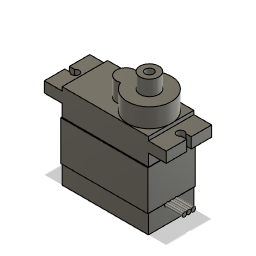
CAM v42 (Autodesk Fusion 360 archive; units mm, degrees)
design "MG90_Rebuild"
Autodesk Fusion 360 part; units mm, degrees
note: some values were not read from the file. Chosen so that the rebuilt part matches the saved one: which face or edge a step refers to. Set by a fixed rule: which sketch regions a step uses.
sketch "ServoRotatingPlate" plane through (0, 0, 0) normal (0, 1, 0) x (1, 0, 0)
  circle A0 centre (0, 0) radius 5.8
  line L0 (5.75, 6) -> (-17.05, 6)
  line L1 (-17.05, 6) -> (-17.05, -6)
  line L2 (-17.05, -6) -> (5.75, -6)
  line L3 (5.75, -6) -> (5.75, 6)
  line L4 (-8.7, 0) -> (5.75, 0) construction
  circle A1 centre (-6.2, 0) radius 2.5
  circle A2 centre (0, 0) radius 2.5
  circle A3 centre (0, 0) radius 1.1
  point P0 (5.8, 0)
  dimension "d4" = 11.6
  dimension "d6" = 12
  dimension "d7" = 22.8
  dimension "d10" = 5
  dimension "d12" = 14.5
  dimension "d13" = 5.75
  dimension "d14" = 8.35
  dimension "d48" = 5
  dimension "d49" = 1.4
  constraint coincident A0.centre A2.centre
  constraint horizontal L0
  constraint vertical L1
  constraint horizontal L2
  constraint vertical L3
  constraint horizontal L4
  constraint midpoint L3 L4.end
  constraint coincident L4 A1.centre
  constraint coincident L4.start A1
  constraint coincident A0.centre L4
  constraint coincident L4 P0
  constraint coincident A0 P0
  constraint concentric A0 A2
  constraint concentric A2 A3
  measures "d4" diameter of A0
  measures "d6" distance of L0.start L2.end
  measures "d7" distance of L0.start L0.end
  measures "d10" diameter of A1
  measures "d12" distance of L4.start P0
  measures "d13" distance of A0.centre L3
  measures "d14" distance of L1 L4.start
  measures "d48" diameter of A2
  measures "d49" distance of A2 A3
extrude "Extrude1" add sketch "ServoRotatingPlate" against normal blind 5 contours A0 L3 | A0 L3 A1 | A0 A1 | A0 A1 | A2 | A3
extrude "Extrude2" add sketch "ServoRotatingPlate" against normal blind 22.5 from surface at -5 contours A0 L3 A1 | A0 L0 L1 L2 L3 A1 | A0 A1 | A0 A1 | A2 | A3
ref_plane "WorkPlane1" through (-5.65, -6, 0) normal (0, 1, 0) x (0, 0, 1)
sketch "EarBase" plane through (-5.65, -6, 0) normal (0, 1, 0) x (1, 0, 0)
  line L0 (16.1, 6) -> (-16.1, 6)
  line L1 (-16.1, 6) -> (-16.1, -6)
  line L2 (-16.1, -6) -> (16.1, -6)
  line L3 (16.1, -6) -> (16.1, 6)
  line L4 (16.1, 6) -> (-16.1, -6) construction
  line L5 (-16.1, 6) -> (16.1, -6) construction
  line L6 (-16.1, 0) -> (16.1, 0) construction
  circle A0 centre (-13.9, 0) radius 1
  line L7 (-14.7, 0.6) -> (-16.1, 0.6)
  line L8 (-14.7, -0.6) -> (-16.1, -0.6)
  line L9 (-11.4, 6) -> (-11.4, -6)
  line L10 (0, 0) -> (0, 6) construction
  line L11 (14.7, 0.6) -> (16.1, 0.6)
  circle A1 centre (13.9, 0) radius 1
  line L12 (14.7, -0.6) -> (16.1, -0.6)
  point P0 (11.4, 6)
  dimension "d26" = 32.2
  dimension "d31" = 2
  dimension "d33" = 1.2
  dimension "d34" = 2.5
  dimension "d35" = 4.7
  constraint perpendicular L0 L1
  constraint parallel L0 L2
  constraint parallel L1 L3
  constraint horizontal L0
  constraint coincident L4 L10.start
  constraint coincident L5 L10.start
  constraint coincident L10.start origin
  constraint coincident L0 P0
  constraint midpoint L1 L6.start
  constraint midpoint L3 L6.end
  constraint coincident L6 A0.centre
  constraint coincident A0 L7.start
  constraint coincident L1 L7.end
  constraint perpendicular L1 L7
  constraint symmetric L6 L7.start L8.start
  constraint symmetric L6 L7.end L8.end
  constraint midpoint L0 L10.end
  constraint symmetric A0 L10 A1
  constraint symmetric L7.start L10 L11.start
  constraint symmetric L7.end L10 L11.end
  constraint symmetric L8.start L10 L12.start
  constraint symmetric L8.end L10 L12.end
  measures "d26" distance of L0.start L0.end
  measures "d31" diameter of A0
  measures "d33" distance of L7.end L8.end
  measures "d34" distance of A0.centre L9
  measures "d35" distance of L0.end L9.start
extrude "Extrude3" add sketch "EarBase" against normal blind 2.8 contours L0 L2 L3 L9 L11 A1 L12 | L0 L1 L2 A0 L7 L8 L9
ref_plane "WorkPlane2" through (-5.65, -22.5, 0) normal (0, -1, 0) x (0, 0, -1)
sketch "StickerBase" plane through (-5.65, -22.5, 0) normal (0, -1, 0) x (1, 0, 0)
  line L0 (11.5, -6.25) -> (-11.5, -6.25)
  line L1 (-11.5, -6.25) -> (-11.5, 6.25)
  line L2 (-11.5, 6.25) -> (11.5, 6.25)
  line L3 (11.5, 6.25) -> (11.5, -6.25)
  line L4 (11.5, -6.25) -> (-11.5, 6.25) construction
  line L5 (-11.5, -6.25) -> (11.5, 6.25) construction
  dimension "d42" = 23
  dimension "d43" = 12.5
  constraint perpendicular L0 L1
  constraint parallel L0 L2
  constraint parallel L1 L3
  constraint horizontal L0
  constraint coincident L4 origin
  constraint coincident L5 origin
  measures "d42" distance of L0.start L0.end
  measures "d43" distance of L0.start L2.end
extrude "Extrude4" add sketch "StickerBase" against normal blind 10.5
extrude "Extrude5" add sketch "ServoRotatingPlate" along normal blind 4 contours A2
sketch "WireHardCoded" plane through (5.75, 0, 0) normal (1, 0, 0) x (0, 0, -1)
  line L0 (6, -22.5) -> (-6, -22.5)
  line L1 (-6, -22.5) -> (-6, -27.5)
  line L2 (-6, -27.5) -> (6, -27.5)
  line L3 (6, -27.5) -> (6, -22.5)
  line L4 (-1.75, -23.5) -> (1.75, -23.5) construction
  line L5 (1.75, -23.5) -> (1.75, -22.3333) construction
  line L6 (1.75, -22.3333) -> (-1.75, -22.3333) construction
  line L7 (-1.75, -22.3333) -> (-1.75, -23.5) construction
  line L8 (0, -27.5) -> (0, -23.5) construction
  line L9 (-1.75, -22.9167) -> (1.75, -22.9167) construction
  circle A0 centre (0, -22.9167) radius 0.5833
  circle A1 centre (-1.17, -22.9167) radius 0.5833
  circle A2 centre (1.17, -22.9167) radius 0.5833
  dimension "d52" = 1.1667
  dimension "d53" = 3.5
  dimension "d54" = 4
  dimension "d57" = 1.17
  dimension "d58" = 0
  constraint horizontal L4
  constraint vertical L5
  constraint horizontal L6
  constraint vertical L7
  constraint midpoint L2 L8.start
  constraint midpoint L4 L8.end
  constraint vertical L8
  constraint midpoint L7 L9.start
  constraint midpoint L5 L9.end
  constraint midpoint L9 A0.centre
  constraint tangent L6 A0
  measures "d52" distance of L4.end L5.end
  measures "d53" distance of L4.start L4.end
  measures "d54" distance of L8.start L8.end
extrude "Extrude6" add sketch "WireHardCoded" along normal up to surface (4.7 mm away) contours L0 A2 | L0 A2 | L0 A0 | L0 A0 | L0 A1 | L0 A1
equation "Note0 = 0" comment "The [0,0,0] is placed at the servo shaft base plane, for better alignment"
equation "Note1 = 1" comment "Improvement for https://www.thingiverse.com/thing:2641076"
equation "BaseCircleD = 11.6 mm"
equation "d4 = BaseCircleD"
equation "BaseRectW = 12 mm"
equation "d6 = BaseRectW"
equation "d7 = BaseRectH"
equation "BaseRectH = 22.8 mm"
equation "BaseCircle2D = 5 mm"
equation "d10 = BaseCircle2D"
equation "E2EDist = 14.5 mm"
equation "d12 = E2EDist"
equation "d13 = CenterMeasureL"
equation "CenterMeasureL = 5.75 mm"
equation "GearIsleHeight = 5 mm"
equation "d17 = -GearIsleHeight"
equation "BoxHeight = 22.5 mm"
equation "d21 = -BoxHeight"
equation "Ear_Down = 1 mm"
equation "d24 = -Ear_Down"
equation "Ear_L = 32.2 mm"
equation "d26 = Ear_L"
equation "Ear_Thick = 2.8 mm"
equation "d28 = -Ear_Thick"
equation "EarScrew_D = 2 mm"
equation "d31 = EarScrew_D"
equation "Ear_Slit = 1.2 mm"
equation "d33 = Ear_Slit"
equation "d34 = HolePos"
equation "HolePos = 2.5 mm"
equation "sticker_height = 10.5 mm"
equation "stick_pos = 5 mm"
equation "d39 = -stick_pos"
equation "Sticker_Profile_L = 23 mm"
equation "Sticker_Profile_W = 12.5 mm"
equation "d42 = Sticker_Profile_L"
equation "d43 = Sticker_Profile_W"
equation "d44 = -sticker_height"
equation "ServoShaftProf = 5 mm"
equation "ServoProfHeight = 4 mm"
equation "d48 = ServoShaftProf"
equation "d50 = ServoProfHeight"
equation "d52 = ( 3.5 / 3 ) * 1 mm"
named bodies: "WireHardCoded"

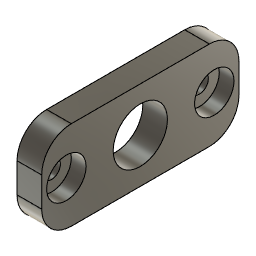
design "mil_tutucu"
Autodesk Fusion 360 part; units mm, degrees
sketch "Sketch1" plane through (0, 0, 0) normal (1, 0, 0) x (0, 1, 0)
  line L0 (0, 0) -> (40, 0)
  line L1 (40, 0) -> (40, 18)
  line L2 (40, 18) -> (0, 18)
  line L3 (0, 18) -> (0, 0)
  circle A0 centre (20, 9) radius 5.5
  line L4 (0, 9) -> (40, 9) construction
  dimension "d1" = 18
  dimension "d2" = 40
  dimension "d3" = 11
  constraint horizontal L0
  constraint vertical L1
  constraint horizontal L2
  constraint vertical L3
  constraint coincident L0.start L3.end
  constraint midpoint L3 L4.start
  constraint midpoint L1 L4.end
  constraint midpoint A0.centre L4
  measures "d1" distance of L0.end L1.end
  measures "d2" distance of L1.end L2.end
  measures "d3" diameter of A0
extrude "Extrude1" add sketch "Sketch1" along normal blind 5
fillet "Fillet1" radius 6 4 edges at (2.5, 0, 18) (2.5, 0, 0) (2.5, 40, 0) (2.5, 40, 18)
sketch "Sketch2" plane through (5, 0, 0) normal (1, 0, 0) x (0, 1, 0)
  circle A0 centre (20, 9) radius 5.5
  arc A1 (40, 12) -> (34, 18) centre (34, 12) ccw
  line L0 (34, 18) -> (6, 18)
  arc A2 (6, 18) -> (0, 12) centre (6, 12) ccw
  line L1 (0, 12) -> (0, 6)
  arc A3 (0, 6) -> (6, 0) centre (6, 6) ccw
  line L2 (6, 0) -> (34, 0)
  arc A4 (34, 0) -> (40, 6) centre (34, 6) ccw
  line L3 (40, 6) -> (40, 12)
  line L4 (40, 9) -> (0, 9) construction
  point P0 (5, 9)
  point P1 (35, 9)
  dimension "d8" = 5
  dimension "d9" = 5
  constraint horizontal P0 P1
  constraint midpoint L3 L4.start
  constraint midpoint L1 L4.end
  constraint coincident P1 L4
  measures "d8" distance of P1 L4.start
  measures "d9" distance of P0 L4.end
hole "Hole1" at (5, 5, 9) at (5, 35, 9) direction (-1, 0, 0) diameter 3.6 depth 7 tip angle 118 counterbore diameter 8 counterbore depth 3

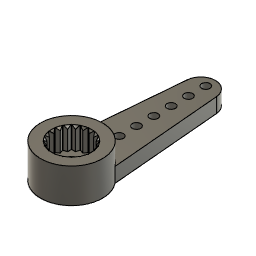
design "MG90_Arm"
Autodesk Fusion 360 part; units mm, degrees
sketch "Arm01Base" plane through (0, 0, 0) normal (0, 1, 0) x (1, 0, 0)
  circle A0 centre (0, 0) radius 3.7
  circle A1 centre (0, 0) radius 2.7
  line L0 (0, -3.7) -> (0, 17.2) construction
  circle A2 centre (0, 15.45) radius 1.75
  line L1 (-1.7434, 15.6016) -> (-2.9, 2.2978)
  line L2 (1.7434, 15.6016) -> (2.9, 2.2978)
  circle A3 centre (0, 0) radius 1.375
  circle A4 centre (0, 16.05) radius 0.5
  circle A5 centre (0, 13.98) radius 0.5
  circle A6 centre (0, 11.91) radius 0.5
  circle A7 centre (0, 9.84) radius 0.5
  circle A8 centre (0, 7.77) radius 0.5
  circle A9 centre (0, 5.7) radius 0.5
  point P0 (0, 16.55)
  dimension "d2" = 7.4
  dimension "d3" = 1
  dimension "d4" = 20.9
  dimension "d5" = 3.5
  dimension "d6" = 2.9
  dimension "d7" = 2.75
  dimension "d8" = 1
  dimension "d9" = 0.65
  dimension "d12" = 0
  dimension "d13" = -10.35
  constraint coincident A0.centre A1.centre
  constraint coincident A0 L0.start
  constraint vertical L0
  constraint coincident A0.centre L0
  constraint coincident L0 A2.centre
  constraint coincident L0.end A2
  constraint coincident A2 L1.start
  constraint coincident A0 L1.end
  constraint tangent A2 L1
  constraint symmetric L0 L1.start L2.start
  constraint symmetric L0 L1.end L2.end
  constraint concentric A1 A3
  constraint coincident L0 A4.centre
  constraint coincident A4 P0
  constraint coincident L0 P0
  measures "d2" diameter of A0
  measures "d3" distance of A0 A1
  measures "d4" distance of L0.start L0.end
  measures "d5" diameter of A2
  measures "d6" distance of L0 L1.end
  measures "d7" diameter of A3
  measures "d8" diameter of A4
  measures "d9" distance of L0.end P0
extrude "Extrude1" add sketch "Arm01Base" along normal blind 1.75 contours A0 | A0 A2 L1 L2 A5 | A2 A5 picked at (0.7406, 14.9094) makes body 1
extrude "Extrude2" add sketch "Arm01Base" along normal blind 4.1 contours A0 bodies 1
ref_plane "WorkPlane1" through (0, 1.5, 0) normal (0, 1, 0) x (0, 0, 1)
extrude "Extrude3" add sketch "Arm01Base" against normal blind 0.5 from surface at 1.5 contours A1 bodies 1
sketch "Teeth01" plane through (0, 1.5, 0) normal (0, 1, 0) x (1, 0, 0)
  circle A0 centre (0, 0) radius 2.1 construction
  circle A1 centre (0, 0) radius 2.4 construction
  line L0 (0, 0) -> (0, 2.4) construction
  line L1 (-0.35, 2.3743) -> (0, 2.1)
  line L2 (0.35, 2.3743) -> (0, 2.1)
  line L3 (-1.0666, 2.15) -> (-0.6489, 1.9972)
  line L4 (-0.4008, 2.3663) -> (-0.6489, 1.9972)
  line L5 (-1.6788, 1.7152) -> (-1.2343, 1.6989)
  line L6 (-1.1124, 2.1266) -> (-1.2343, 1.6989)
  line L7 (-2.1266, 1.1124) -> (-1.6989, 1.2343)
  line L8 (-1.7152, 1.6788) -> (-1.6989, 1.2343)
  line L9 (-2.3663, 0.4008) -> (-1.9972, 0.6489)
  line L10 (-2.15, 1.0666) -> (-1.9972, 0.6489)
  line L11 (-2.3743, -0.35) -> (-2.1, 0)
  line L12 (-2.3743, 0.35) -> (-2.1, 0)
  line L13 (-2.15, -1.0666) -> (-1.9972, -0.6489)
  line L14 (-2.3663, -0.4008) -> (-1.9972, -0.6489)
  line L15 (-1.7152, -1.6788) -> (-1.6989, -1.2343)
  line L16 (-2.1266, -1.1124) -> (-1.6989, -1.2343)
  line L17 (-1.1124, -2.1266) -> (-1.2343, -1.6989)
  line L18 (-1.6788, -1.7152) -> (-1.2343, -1.6989)
  line L19 (-0.4008, -2.3663) -> (-0.6489, -1.9972)
  line L20 (-1.0666, -2.15) -> (-0.6489, -1.9972)
  line L21 (0.35, -2.3743) -> (0, -2.1)
  line L22 (-0.35, -2.3743) -> (0, -2.1)
  line L23 (1.0666, -2.15) -> (0.6489, -1.9972)
  line L24 (0.4008, -2.3663) -> (0.6489, -1.9972)
  line L25 (1.6788, -1.7152) -> (1.2343, -1.6989)
  line L26 (1.1124, -2.1266) -> (1.2343, -1.6989)
  line L27 (2.1266, -1.1124) -> (1.6989, -1.2343)
  line L28 (1.7152, -1.6788) -> (1.6989, -1.2343)
  line L29 (2.3663, -0.4008) -> (1.9972, -0.6489)
  line L30 (2.15, -1.0666) -> (1.9972, -0.6489)
  line L31 (2.3743, 0.35) -> (2.1, 0)
  line L32 (2.3743, -0.35) -> (2.1, 0)
  line L33 (2.15, 1.0666) -> (1.9972, 0.6489)
  line L34 (2.3663, 0.4008) -> (1.9972, 0.6489)
  line L35 (1.7152, 1.6788) -> (1.6989, 1.2343)
  line L36 (2.1266, 1.1124) -> (1.6989, 1.2343)
  line L37 (1.1124, 2.1266) -> (1.2343, 1.6989)
  line L38 (1.6788, 1.7152) -> (1.2343, 1.6989)
  line L39 (0.4008, 2.3663) -> (0.6489, 1.9972)
  line L40 (1.0666, 2.15) -> (0.6489, 1.9972)
  circle A2 centre (0, 0) radius 2.7
  circle A3 centre (0, 0) radius 2.4
  dimension "d22" = 4.2
  dimension "d23" = 4.8
  dimension "d24" = 0.35
  dimension "d26" = 360
  constraint coincident A0.centre A1.centre
  constraint concentric A0 A1
  constraint coincident A1 L0.end
  constraint vertical L0
  constraint coincident A1 L1.start
  constraint coincident A0 L1.end
  constraint coincident L0 L1.end
  constraint coincident A1 L2.start
  constraint symmetric L0 L1.start L2.start
  constraint coincident L39.start A3
  measures "d22" diameter of A0
  measures "d23" diameter of A1
  measures "d24" horizontal distance of L0.end L2.start
extrude "Extrude4" add sketch "Teeth01" along normal up to surface (2.6 mm away) contours L1 L2 A3 | L3 L4 A3 | L39 L40 A3 | L5 L6 A3 | L37 L38 A3 | L7 L8 A3 | L35 L36 A3 | L9 L10 A3 | L33 L34 A3 | L11 L12 A3 | L31 L32 A3 | L13 L14 A3 | L29 L30 A3 | L15 L16 A3 | L27 L28 A3 | L17 L18 A3 | L25 L26 A3 | L19 L20 A3 | L23 L24 A3 | L21 L22 A3 | A2 bodies 1
sketch "TeethChamfer01" plane through (0, 0, 0) normal (1, 0, 0) x (0, 0, -1)
  line L0 (3.7, 4.1) -> (-3.7, 4.1) construction
  line L1 (0, 0) -> (0, 4.1) construction
  line L2 (2.3743, 4.1) -> (2.1, 3.8)
  line L3 (2.1, 3.8) -> (2.1, 4.1)
  line L4 (2.3743, 4.1) -> (2.1, 4.1)
  point P0 (2.3743, 4.1)
  point P1 (2.1, 4.1)
  dimension "d29" = 0.3
  constraint coincident L1.start origin
  constraint midpoint L0 L1.end
  constraint coincident P0 L2.start
  constraint coincident L0 P1
  constraint perpendicular L0 L3
  constraint coincident P1 L3.end
  measures "d29" distance of L2.end P1
revolve "Revolve1" cut sketch "TeethChamfer01" angle 360 about axis through (0, 0, 0) along (0, 1, 0) bodies 1
copy_body "Body->Comp1" bodies 1 removing the originals makes body 2 in component "Arm01"
sketch "Arm02Base" plane through (0, 0, 0) normal (0, 1, 0) x (1, 0, 0)
  line L0 (0, 0) -> (30, 0) construction
  circle A0 centre (30, 0) radius 3.45
  circle A1 centre (30, 0) radius 2.25
  line L1 (30, -15.675) -> (30, 15.675) construction
  circle A2 centre (30, 13.925) radius 1.75
  line L2 (28.2556, 14.0649) -> (27.3, 2.1477)
  line L3 (31.7444, 14.0649) -> (32.7, 2.1477)
  circle A3 centre (30, 14.375) radius 0.5
  circle A4 centre (30, 12.405) radius 0.5
  circle A5 centre (30, 10.435) radius 0.5
  circle A6 centre (30, 8.465) radius 0.5
  circle A7 centre (30, 6.495) radius 0.5
  circle A8 centre (30, 4.525) radius 0.5
  line L4 (31.7444, -14.0649) -> (32.7, -2.1477)
  circle A9 centre (30, -13.925) radius 1.75
  circle A10 centre (30, -12.405) radius 0.5
  circle A11 centre (30, -10.435) radius 0.5
  circle A12 centre (30, -8.465) radius 0.5
  circle A13 centre (30, -6.495) radius 0.5
  circle A14 centre (30, -4.525) radius 0.5
  line L5 (28.2556, -14.0649) -> (27.3, -2.1477)
  circle A15 centre (30, -14.375) radius 0.5
  circle A16 centre (30, 0) radius 1.25
  point P0 (30, 14.875)
  dimension "d31" = 30
  dimension "d32" = 6.9
  dimension "d33" = 1.2
  dimension "d34" = 31.35
  dimension "d35" = 3.5
  dimension "d36" = 2.7
  dimension "d37" = 1
  dimension "d38" = 0.8
  dimension "d41" = 0
  dimension "d42" = -9.85
  dimension "d47" = 2.5
  constraint coincident L0.start origin
  constraint horizontal L0
  constraint coincident L0.end A0.centre
  constraint concentric A0 A1
  constraint perpendicular L0 L1
  constraint coincident L1 A2.centre
  constraint coincident L1.end A2
  constraint midpoint L0.end L1
  constraint coincident A2 L2.start
  constraint coincident A0 L2.end
  constraint tangent A2 L2
  constraint symmetric L1 L2.start L3.start
  constraint symmetric L1 L2.end L3.end
  constraint coincident L1 A3.centre
  constraint coincident A3 P0
  constraint coincident L1 P0
  constraint symmetric L0 A2 A9
  constraint symmetric L0 L2.start L5.start
  constraint symmetric L0 L2.end L5.end
  constraint symmetric L0 L3.start L4.start
  constraint symmetric L0 L3.end L4.end
  constraint symmetric L0 A4 A10
  constraint symmetric L0 A5 A11
  constraint symmetric L0 A6 A12
  constraint symmetric L0 A7 A13
  constraint symmetric L0 A8 A14
  constraint symmetric L0 A3 A15
  constraint concentric A0 A16
  measures "d31" distance of L0.start L0.end
  measures "d32" diameter of A0
  measures "d33" distance of A0 A1
  measures "d34" distance of L1.start L1.end
  measures "d35" diameter of A2
  measures "d36" distance of L1 L2.end
  measures "d37" diameter of A3
  measures "d38" distance of L1.end P0
  measures "d47" diameter of A16
component "Arm01" placed x (1, 0, 0) y (0, 1, 0) z (0, 0, 1) at (0, 0, 0)
equation "SA1_Hull_D = 7.4 mm"
equation "d2 = SA1_Hull_D"
equation "d6 = ( 5.8 / 2 ) * 1 mm"
equation "d36 = ( 5.4 / 2 ) * 1 mm"
named bodies: "Arm01"

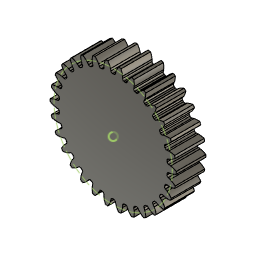
design "smallgear"
description: Spur Gear; Module: 1.000000; Number of Teeth: 30; Pressure Angle: 20.000000; Root Fillet Radius: 0.040000; Clearance: 0.010000; Gear Thickness: 0.750000; Hole Diameter: 0.000000;
Autodesk Fusion 360 part; units mm, degrees
sketch "sketch 24713" plane through (0, 0, 0) normal (0, 1, 0) x (1, 0, 0)
  spline S0 degree 3 poles (8.0197, -12.2129) (7.9317, -11.9434) (7.8522, -11.7971) (7.8241, -11.7495) knots 0 0 0 0 1 1 1 1
  spline S1 degree 3 poles (10.9388, -11.678) (10.7651, -11.0274) (10.5532, -10.5719) (10.3836, -10.2786) knots 0 0 0 0 1 1 1 1
  spline S2 degree 3 poles (8.7567, -11.072) (8.7932, -11.1134) (8.9078, -11.2342) (9.1369, -11.4012) knots 0 0 0 0 1 1 1 1
  arc A0 (10.4706, -12.0996) -> (10.9388, -11.678) centre (0, 0) ccw
  spline S3 degree 3 poles (10.3836, -10.2786) (10.2415, -10.0333) (10.1333, -9.9067) (10.096, -9.866) knots 0 0 0 0 1 1 1 1
  arc A1 (10.8673, -9.0094) -> (10.3337, -9.0707) centre (10.6343, -9.3345) ccw
  spline S4 degree 3 poles (10.8673, -9.0094) (10.9117, -9.0423) (11.0489, -9.1366) (11.3077, -9.2524) knots 0 0 0 0 1 1 1 1
  spline S5 degree 3 poles (9.1369, -11.4012) (9.4109, -11.6005) (9.8417, -11.8588) (10.4706, -12.0996) knots 0 0 0 0 1 1 1 1
  arc A2 (11.82, -7.025) -> (11.9938, -6.7239) centre (0, 0) ccw
  spline S6 degree 3 poles (12.503, -6.5531) (12.5532, -6.576) (12.707, -6.6398) (12.9842, -6.6992) knots 0 0 0 0 1 1 1 1
  arc A3 (14.4867, -6.7947) -> (14.743, -6.2191) centre (0, 0) ccw
  arc A4 (10.1011, -9.329) -> (10.3337, -9.0707) centre (0, 0) ccw
  arc A5 (12.503, -6.5531) -> (11.9938, -6.7239) centre (12.3427, -6.9196) ccw
  spline S7 degree 3 poles (12.9842, -6.6992) (13.3156, -6.7698) (13.8143, -6.8306) (14.4867, -6.7947) knots 0 0 0 0 1 1 1 1
  arc A6 (13.0223, -4.4139) -> (13.236, -4.9067) centre (13.4011, -4.5423) ccw
  spline S8 degree 3 poles (14.743, -6.2191) (14.3197, -5.6954) (13.9408, -5.3655) (13.6666, -5.1666) knots 0 0 0 0 1 1 1 1
  spline S9 degree 3 poles (13.6666, -5.1666) (13.437, -5.0003) (13.2867, -4.9286) (13.236, -4.9067) knots 0 0 0 0 1 1 1 1
  arc A7 (13.5922, -3.8104) -> (13.1297, -4.0834) centre (13.5116, -4.2022) ccw
  spline S10 degree 3 poles (12.2938, -7.8951) (12.1037, -7.6847) (11.9716, -7.5834) (11.9266, -7.5514) knots 0 0 0 0 1 1 1 1
  arc A8 (10.1011, -9.329) -> (10.096, -9.866) centre (10.395, -9.6003) ccw
  spline S11 degree 3 poles (11.3077, -9.2524) (11.6171, -9.3904) (12.0922, -9.5535) (12.7574, -9.6582) knots 0 0 0 0 1 1 1 1
  spline S12 degree 3 poles (13.1278, -9.1485) (12.8226, -8.5482) (12.5206, -8.1467) (12.2938, -7.8951) knots 0 0 0 0 1 1 1 1
  arc A9 (12.7574, -9.6582) -> (13.1278, -9.1485) centre (0, 0) ccw
  arc A10 (11.82, -7.025) -> (11.9266, -7.5514) centre (12.1639, -7.2293) ccw
  arc A11 (13.6554, -1.61) -> (13.9669, -2.0475) centre (14.0527, -1.6568) ccw
  spline S13 degree 3 poles (3.4962, -13.6764) (3.5128, -13.7291) (3.5684, -13.8861) (3.7097, -14.1318) knots 0 0 0 0 1 1 1 1
  arc A12 (2.6886, -13.4846) -> (2.3687, -13.9161) centre (2.7668, -13.8769) ccw
  spline S14 degree 3 poles (3.7097, -14.1318) (3.8789, -14.4253) (4.1674, -14.8366) (4.644, -15.3123) knots 0 0 0 0 1 1 1 1
  spline S15 degree 3 poles (14.4421, -2.2122) (14.183, -2.0973) (14.0211, -2.0585) (13.9669, -2.0475) knots 0 0 0 0 1 1 1 1
  spline S16 degree 3 poles (14.0933, -3.8532) (14.4321, -3.8534) (14.9325, -3.8092) (15.5828, -3.6343) knots 0 0 0 0 1 1 1 1
  spline S17 degree 3 poles (15.7138, -3.018) (15.1909, -2.5937) (14.7517, -2.3498) (14.4421, -2.2122) knots 0 0 0 0 1 1 1 1
  spline S18 degree 3 poles (13.5922, -3.8104) (13.6461, -3.8224) (13.8098, -3.8527) (14.0933, -3.8532) knots 0 0 0 0 1 1 1 1
  arc A13 (2.6886, -13.4846) -> (3.0285, -13.4123) centre (0, 0) ccw
  arc A14 (13.0223, -4.4139) -> (13.1297, -4.0834) centre (0, 0) ccw
  arc A15 (15.5828, -3.6343) -> (15.7138, -3.018) centre (0, 0) ccw
  arc A16 (4.644, -15.3123) -> (5.2432, -15.1176) centre (0, 0) ccw
  arc A17 (3.4962, -13.6764) -> (3.0285, -13.4123) centre (3.1166, -13.8025) ccw
  spline S19 degree 3 poles (2.3589, -14.4189) (2.3881, -14.1369) (2.375, -13.9709) (2.3687, -13.9161) knots 0 0 0 0 1 1 1 1
  spline S20 degree 3 poles (8.0197, 12.2129) (8.1246, 12.535) (8.2372, 13.0246) (8.2718, 13.6971) knots 0 0 0 0 1 1 1 1
  spline S21 degree 3 poles (7.7261, 14.0121) (7.161, 13.6459) (6.7933, 13.3036) (6.5668, 13.0517) knots 0 0 0 0 1 1 1 1
  arc A18 (5.7509, 12.4896) -> (6.2633, 12.6506) centre (5.9182, 12.8529) ccw
  arc A19 (13.6917, 1.2643) -> (13.6554, 1.61) centre (0, 0) ccw
  spline S22 degree 3 poles (11.9266, 7.5514) (11.9716, 7.5834) (12.1037, 7.6847) (12.2938, 7.8951) knots 0 0 0 0 1 1 1 1
  arc A20 (5.2103, 13.1195) -> (5.4334, 12.6309) centre (5.5915, 12.9984) ccw
  spline S23 degree 3 poles (5.2103, 13.1195) (5.2279, 13.1718) (5.2752, 13.3315) (5.3052, 13.6134) knots 0 0 0 0 1 1 1 1
  spline S24 degree 3 poles (14.5865, -0.8388) (14.9179, -0.7686) (15.3982, -0.6213) (15.9979, -0.315) knots 0 0 0 0 1 1 1 1
  spline S25 degree 3 poles (13.6666, 5.1666) (13.9408, 5.3655) (14.3197, 5.6954) (14.743, 6.2191) knots 0 0 0 0 1 1 1 1
  spline S26 degree 3 poles (5.3052, 13.6134) (5.3409, 13.9503) (5.3492, 14.4526) (5.2432, 15.1176) knots 0 0 0 0 1 1 1 1
  spline S27 degree 3 poles (14.5865, 0.8388) (14.3091, 0.8973) (14.1426, 0.9017) (14.0874, 0.9011) knots 0 0 0 0 1 1 1 1
  spline S28 degree 3 poles (12.2938, 7.8951) (12.5206, 8.1467) (12.8226, 8.5482) (13.1278, 9.1485) knots 0 0 0 0 1 1 1 1
  spline S29 degree 3 poles (4.644, 15.3123) (4.1674, 14.8366) (3.8789, 14.4253) (3.7097, 14.1318) knots 0 0 0 0 1 1 1 1
  spline S30 degree 3 poles (6.5668, 13.0517) (6.3774, 12.8407) (6.2905, 12.6987) (6.2633, 12.6506) knots 0 0 0 0 1 1 1 1
  spline S31 degree 3 poles (2.3687, 13.9161) (2.375, 13.9709) (2.3881, 14.1369) (2.3589, 14.4189) knots 0 0 0 0 1 1 1 1
  spline S32 degree 3 poles (15.5828, 3.6343) (14.9325, 3.8092) (14.4321, 3.8534) (14.0933, 3.8532) knots 0 0 0 0 1 1 1 1
  arc A21 (2.3687, 13.9161) -> (2.6886, 13.4846) centre (2.7668, 13.8769) ccw
  arc A22 (3.0285, 13.4123) -> (3.4962, 13.6764) centre (3.1166, 13.8025) ccw
  spline S33 degree 3 poles (3.7097, 14.1318) (3.5684, 13.8861) (3.5128, 13.7291) (3.4962, 13.6764) knots 0 0 0 0 1 1 1 1
  arc A23 (3.0285, 13.4123) -> (2.6886, 13.4846) centre (0, 0) ccw
  spline S34 degree 3 poles (2.3589, 14.4189) (2.3237, 14.7559) (2.2275, 15.2489) (1.9855, 15.8773) knots 0 0 0 0 1 1 1 1
  arc A24 (1.9855, 15.8773) -> (1.3589, 15.9432) centre (0, 0) ccw
  arc A25 (0.1738, 13.7489) -> (0.5763, 14.1044) centre (0.1788, 14.1489) ccw
  arc A26 (10.3337, 9.0707) -> (10.1011, 9.329) centre (0, 0) ccw
  arc A27 (11.9266, 7.5514) -> (11.82, 7.025) centre (12.1639, 7.2293) ccw
  arc A28 (15.9979, -0.315) -> (15.9979, 0.315) centre (0, 0) ccw
  spline S35 degree 3 poles (14.4421, 2.2122) (14.7517, 2.3498) (15.1909, 2.5937) (15.7138, 3.018) knots 0 0 0 0 1 1 1 1
  spline S36 degree 3 poles (11.3077, 9.2524) (11.0489, 9.1366) (10.9117, 9.0423) (10.8673, 9.0094) knots 0 0 0 0 1 1 1 1
  arc A29 (13.6917, 1.2643) -> (14.0874, 0.9011) centre (14.0901, 1.3011) ccw
  arc A30 (13.1297, 4.0834) -> (13.0223, 4.4139) centre (0, 0) ccw
  arc A31 (13.9669, 2.0475) -> (13.6554, 1.61) centre (14.0527, 1.6568) ccw
  arc A32 (13.6554, -1.61) -> (13.6917, -1.2643) centre (0, 0) ccw
  arc A33 (13.236, 4.9067) -> (13.0223, 4.4139) centre (13.4011, 4.5423) ccw
  arc A34 (11.9938, 6.7239) -> (12.503, 6.5531) centre (12.3427, 6.9196) ccw
  arc A35 (7.8241, 11.7495) -> (7.9408, 11.2252) centre (8.1718, 11.5518) ccw
  spline S37 degree 3 poles (13.236, 4.9067) (13.2867, 4.9286) (13.437, 5.0003) (13.6666, 5.1666) knots 0 0 0 0 1 1 1 1
  spline S38 degree 3 poles (14.4867, 6.7947) (13.8143, 6.8306) (13.3156, 6.7698) (12.9842, 6.6992) knots 0 0 0 0 1 1 1 1
  spline S39 degree 3 poles (13.9669, 2.0475) (14.0211, 2.0585) (14.183, 2.0973) (14.4421, 2.2122) knots 0 0 0 0 1 1 1 1
  arc A36 (11.9938, 6.7239) -> (11.82, 7.025) centre (0, 0) ccw
  arc A37 (10.3337, 9.0707) -> (10.8673, 9.0094) centre (10.6343, 9.3345) ccw
  arc A38 (10.096, 9.866) -> (10.1011, 9.329) centre (10.395, 9.6003) ccw
  arc A39 (15.7138, 3.018) -> (15.5828, 3.6343) centre (0, 0) ccw
  spline S40 degree 3 poles (12.9842, 6.6992) (12.707, 6.6398) (12.5532, 6.576) (12.503, 6.5531) knots 0 0 0 0 1 1 1 1
  arc A40 (10.9388, 11.678) -> (10.4706, 12.0996) centre (0, 0) ccw
  arc A41 (8.222, 11.0209) -> (7.9408, 11.2252) centre (0, 0) ccw
  arc A42 (13.1278, 9.1485) -> (12.7574, 9.6582) centre (0, 0) ccw
  arc A43 (14.743, 6.2191) -> (14.4867, 6.7947) centre (0, 0) ccw
  spline S41 degree 3 poles (9.1369, 11.4012) (8.9078, 11.2342) (8.7932, 11.1134) (8.7567, 11.072) knots 0 0 0 0 1 1 1 1
  spline S42 degree 3 poles (10.3836, 10.2786) (10.5532, 10.5719) (10.7651, 11.0274) (10.9388, 11.678) knots 0 0 0 0 1 1 1 1
  arc A44 (8.222, 11.0209) -> (8.7567, 11.072) centre (8.4612, 11.3416) ccw
  arc A45 (14.0874, -0.9011) -> (13.6917, -1.2643) centre (14.0901, -1.3011) ccw
  spline S43 degree 3 poles (10.4706, 12.0996) (9.8417, 11.8588) (9.4109, 11.6005) (9.1369, 11.4012) knots 0 0 0 0 1 1 1 1
  arc A46 (13.1297, 4.0834) -> (13.5922, 3.8104) centre (13.5116, 4.2022) ccw
  spline S44 degree 3 poles (14.0874, -0.9011) (14.1426, -0.9017) (14.3091, -0.8973) (14.5865, -0.8388) knots 0 0 0 0 1 1 1 1
  spline S45 degree 3 poles (12.7574, 9.6582) (12.0922, 9.5535) (11.6171, 9.3904) (11.3077, 9.2524) knots 0 0 0 0 1 1 1 1
  arc A47 (8.2718, 13.6971) -> (7.7261, 14.0121) centre (0, 0) ccw
  spline S46 degree 3 poles (7.8241, 11.7495) (7.8522, 11.7971) (7.9317, 11.9434) (8.0197, 12.2129) knots 0 0 0 0 1 1 1 1
  arc A48 (5.2432, 15.1176) -> (4.644, 15.3123) centre (0, 0) ccw
  arc A49 (5.7509, 12.4896) -> (5.4334, 12.6309) centre (0, 0) ccw
  spline S47 degree 3 poles (15.9979, 0.315) (15.3982, 0.6213) (14.9179, 0.7686) (14.5865, 0.8388) knots 0 0 0 0 1 1 1 1
  spline S48 degree 3 poles (14.0933, 3.8532) (13.8098, 3.8527) (13.6461, 3.8224) (13.5922, 3.8104) knots 0 0 0 0 1 1 1 1
  spline S49 degree 3 poles (10.096, 9.866) (10.1333, 9.9067) (10.2415, 10.0333) (10.3836, 10.2786) knots 0 0 0 0 1 1 1 1
  arc A50 (-7.9408, 11.2252) -> (-8.222, 11.0209) centre (0, 0) ccw
  arc A51 (-12.7574, 9.6582) -> (-13.1278, 9.1485) centre (0, 0) ccw
  arc A52 (-11.82, 7.025) -> (-11.9938, 6.7239) centre (0, 0) ccw
  spline S50 degree 3 poles (-14.743, 6.2191) (-14.3197, 5.6954) (-13.9408, 5.3655) (-13.6666, 5.1666) knots 0 0 0 0 1 1 1 1
  arc A53 (-10.4706, 12.0996) -> (-10.9388, 11.678) centre (0, 0) ccw
  arc A54 (-4.644, 15.3123) -> (-5.2432, 15.1176) centre (0, 0) ccw
  spline S51 degree 3 poles (-13.6666, 5.1666) (-13.437, 5.0003) (-13.2867, 4.9286) (-13.236, 4.9067) knots 0 0 0 0 1 1 1 1
  spline S52 degree 3 poles (-2.3589, 14.4189) (-2.3881, 14.1369) (-2.375, 13.9709) (-2.3687, 13.9161) knots 0 0 0 0 1 1 1 1
  arc A55 (-5.4334, 12.6309) -> (-5.7509, 12.4896) centre (0, 0) ccw
  spline S53 degree 3 poles (-8.2718, 13.6971) (-8.2372, 13.0246) (-8.1246, 12.535) (-8.0197, 12.2129) knots 0 0 0 0 1 1 1 1
  arc A56 (-11.82, 7.025) -> (-11.9266, 7.5514) centre (-12.1639, 7.2293) ccw
  arc A57 (-13.5922, 3.8104) -> (-13.1297, 4.0834) centre (-13.5116, 4.2022) ccw
  arc A58 (-1.3589, 15.9432) -> (-1.9855, 15.8773) centre (0, 0) ccw
  arc A59 (-14.0874, 0.9011) -> (-13.6917, 1.2643) centre (-14.0901, 1.3011) ccw
  arc A60 (-13.6554, 1.61) -> (-13.9669, 2.0475) centre (-14.0527, 1.6568) ccw
  spline S54 degree 3 poles (-5.2432, 15.1176) (-5.3492, 14.4526) (-5.3409, 13.9503) (-5.3052, 13.6134) knots 0 0 0 0 1 1 1 1
  arc A61 (-15.9979, 0.315) -> (-15.9979, -0.315) centre (0, 0) ccw
  arc A62 (-7.9408, 11.2252) -> (-7.8241, 11.7495) centre (-8.1718, 11.5518) ccw
  arc A63 (-10.1011, 9.329) -> (-10.3337, 9.0707) centre (0, 0) ccw
  spline S55 degree 3 poles (-10.9388, 11.678) (-10.7651, 11.0274) (-10.5532, 10.5719) (-10.3836, 10.2786) knots 0 0 0 0 1 1 1 1
  spline S56 degree 3 poles (-10.3836, 10.2786) (-10.2415, 10.0333) (-10.1333, 9.9067) (-10.096, 9.866) knots 0 0 0 0 1 1 1 1
  spline S57 degree 3 poles (-14.4421, 2.2122) (-14.183, 2.0973) (-14.0211, 2.0585) (-13.9669, 2.0475) knots 0 0 0 0 1 1 1 1
  spline S58 degree 3 poles (0.6905, 14.5943) (0.6033, 14.3245) (0.5816, 14.1594) (0.5763, 14.1044) knots 0 0 0 0 1 1 1 1
  spline S59 degree 3 poles (-0.6905, 14.5943) (-0.795, 14.9166) (-0.9916, 15.3788) (-1.3589, 15.9432) knots 0 0 0 0 1 1 1 1
  arc A64 (-0.5763, 14.1044) -> (-0.1738, 13.7489) centre (-0.1788, 14.1489) ccw
  spline S60 degree 3 poles (1.3589, 15.9432) (0.9916, 15.3788) (0.795, 14.9166) (0.6905, 14.5943) knots 0 0 0 0 1 1 1 1
  spline S61 degree 3 poles (-1.9855, 15.8773) (-2.2275, 15.2489) (-2.3237, 14.7559) (-2.3589, 14.4189) knots 0 0 0 0 1 1 1 1
  spline S62 degree 3 poles (-8.0197, 12.2129) (-7.9317, 11.9434) (-7.8522, 11.7971) (-7.8241, 11.7495) knots 0 0 0 0 1 1 1 1
  arc A65 (-6.2633, 12.6506) -> (-5.7509, 12.4896) centre (-5.9182, 12.8529) ccw
  arc A66 (-7.7261, 14.0121) -> (-8.2718, 13.6971) centre (0, 0) ccw
  arc A67 (-2.6886, 13.4846) -> (-3.0285, 13.4123) centre (0, 0) ccw
  arc A68 (-10.8673, 9.0094) -> (-10.3337, 9.0707) centre (-10.6343, 9.3345) ccw
  arc A69 (-3.4962, 13.6764) -> (-3.0285, 13.4123) centre (-3.1166, 13.8025) ccw
  spline S63 degree 3 poles (-11.3077, 9.2524) (-11.6171, 9.3904) (-12.0922, 9.5535) (-12.7574, 9.6582) knots 0 0 0 0 1 1 1 1
  spline S64 degree 3 poles (-13.1278, 9.1485) (-12.8226, 8.5482) (-12.5206, 8.1467) (-12.2938, 7.8951) knots 0 0 0 0 1 1 1 1
  spline S65 degree 3 poles (-3.7097, 14.1318) (-3.8789, 14.4253) (-4.1674, 14.8366) (-4.644, 15.3123) knots 0 0 0 0 1 1 1 1
  arc A70 (0.1738, 13.7489) -> (-0.1738, 13.7489) centre (0, 0) ccw
  spline S66 degree 3 poles (-12.503, 6.5531) (-12.5532, 6.576) (-12.707, 6.6398) (-12.9842, 6.6992) knots 0 0 0 0 1 1 1 1
  spline S67 degree 3 poles (-13.5922, 3.8104) (-13.6461, 3.8224) (-13.8098, 3.8527) (-14.0933, 3.8532) knots 0 0 0 0 1 1 1 1
  arc A71 (-12.503, 6.5531) -> (-11.9938, 6.7239) centre (-12.3427, 6.9196) ccw
  arc A72 (-14.4867, 6.7947) -> (-14.743, 6.2191) centre (0, 0) ccw
  spline S68 degree 3 poles (-14.0874, 0.9011) (-14.1426, 0.9017) (-14.3091, 0.8973) (-14.5865, 0.8388) knots 0 0 0 0 1 1 1 1
  spline S69 degree 3 poles (-14.5865, 0.8388) (-14.9179, 0.7686) (-15.3982, 0.6213) (-15.9979, 0.315) knots 0 0 0 0 1 1 1 1
  spline S70 degree 3 poles (-5.3052, 13.6134) (-5.2752, 13.3315) (-5.2279, 13.1718) (-5.2103, 13.1195) knots 0 0 0 0 1 1 1 1
  spline S71 degree 3 poles (-3.4962, 13.6764) (-3.5128, 13.7291) (-3.5684, 13.8861) (-3.7097, 14.1318) knots 0 0 0 0 1 1 1 1
  arc A73 (-5.4334, 12.6309) -> (-5.2103, 13.1195) centre (-5.5915, 12.9984) ccw
  spline S72 degree 3 poles (-6.2633, 12.6506) (-6.2905, 12.6987) (-6.3774, 12.8407) (-6.5668, 13.0517) knots 0 0 0 0 1 1 1 1
  spline S73 degree 3 poles (-12.9842, 6.6992) (-13.3156, 6.7698) (-13.8143, 6.8306) (-14.4867, 6.7947) knots 0 0 0 0 1 1 1 1
  arc A74 (-2.6886, 13.4846) -> (-2.3687, 13.9161) centre (-2.7668, 13.8769) ccw
  spline S74 degree 3 poles (-14.0933, 3.8532) (-14.4321, 3.8534) (-14.9325, 3.8092) (-15.5828, 3.6343) knots 0 0 0 0 1 1 1 1
  arc A75 (-15.5828, 3.6343) -> (-15.7138, 3.018) centre (0, 0) ccw
  arc A76 (-13.0223, 4.4139) -> (-13.236, 4.9067) centre (-13.4011, 4.5423) ccw
  spline S75 degree 3 poles (-10.8673, 9.0094) (-10.9117, 9.0423) (-11.0489, 9.1366) (-11.3077, 9.2524) knots 0 0 0 0 1 1 1 1
  spline S76 degree 3 poles (-15.7138, 3.018) (-15.1909, 2.5937) (-14.7517, 2.3498) (-14.4421, 2.2122) knots 0 0 0 0 1 1 1 1
  spline S77 degree 3 poles (-8.7567, 11.072) (-8.7932, 11.1134) (-8.9078, 11.2342) (-9.1369, 11.4012) knots 0 0 0 0 1 1 1 1
  arc A77 (-13.0223, 4.4139) -> (-13.1297, 4.0834) centre (0, 0) ccw
  spline S78 degree 3 poles (-6.5668, 13.0517) (-6.7933, 13.3036) (-7.161, 13.6459) (-7.7261, 14.0121) knots 0 0 0 0 1 1 1 1
  spline S79 degree 3 poles (-0.5763, 14.1044) (-0.5816, 14.1594) (-0.6033, 14.3245) (-0.6905, 14.5943) knots 0 0 0 0 1 1 1 1
  arc A78 (-10.1011, 9.329) -> (-10.096, 9.866) centre (-10.395, 9.6003) ccw
  spline S80 degree 3 poles (-9.1369, 11.4012) (-9.4109, 11.6005) (-9.8417, 11.8588) (-10.4706, 12.0996) knots 0 0 0 0 1 1 1 1
  spline S81 degree 3 poles (-12.2938, 7.8951) (-12.1037, 7.6847) (-11.9716, 7.5834) (-11.9266, 7.5514) knots 0 0 0 0 1 1 1 1
  arc A79 (-8.7567, 11.072) -> (-8.222, 11.0209) centre (-8.4612, 11.3416) ccw
  arc A80 (-13.9669, -2.0475) -> (-13.6554, -1.61) centre (-14.0527, -1.6568) ccw
  spline S82 degree 3 poles (-11.9266, -7.5514) (-11.9716, -7.5834) (-12.1037, -7.6847) (-12.2938, -7.8951) knots 0 0 0 0 1 1 1 1
  spline S83 degree 3 poles (-8.0197, -12.2129) (-8.1246, -12.535) (-8.2372, -13.0246) (-8.2718, -13.6971) knots 0 0 0 0 1 1 1 1
  arc A81 (-13.1297, -4.0834) -> (-13.5922, -3.8104) centre (-13.5116, -4.2022) ccw
  arc A82 (-2.3687, -13.9161) -> (-2.6886, -13.4846) centre (-2.7668, -13.8769) ccw
  arc A83 (-3.0285, -13.4123) -> (-2.6886, -13.4846) centre (0, 0) ccw
  spline S84 degree 3 poles (-10.4706, -12.0996) (-9.8417, -11.8588) (-9.4109, -11.6005) (-9.1369, -11.4012) knots 0 0 0 0 1 1 1 1
  spline S85 degree 3 poles (-14.5865, -0.8388) (-14.3091, -0.8973) (-14.1426, -0.9017) (-14.0874, -0.9011) knots 0 0 0 0 1 1 1 1
  arc A84 (-13.1278, -9.1485) -> (-12.7574, -9.6582) centre (0, 0) ccw
  arc A85 (-8.222, -11.0209) -> (-7.9408, -11.2252) centre (0, 0) ccw
  spline S86 degree 3 poles (-7.8241, -11.7495) (-7.8522, -11.7971) (-7.9317, -11.9434) (-8.0197, -12.2129) knots 0 0 0 0 1 1 1 1
  spline S87 degree 3 poles (-14.0933, -3.8532) (-13.8098, -3.8527) (-13.6461, -3.8224) (-13.5922, -3.8104) knots 0 0 0 0 1 1 1 1
  arc A86 (-13.6917, -1.2643) -> (-14.0874, -0.9011) centre (-14.0901, -1.3011) ccw
  spline S88 degree 3 poles (-12.7574, -9.6582) (-12.0922, -9.5535) (-11.6171, -9.3904) (-11.3077, -9.2524) knots 0 0 0 0 1 1 1 1
  arc A87 (-1.9855, -15.8773) -> (-1.3589, -15.9432) centre (0, 0) ccw
  arc A88 (-8.2718, -13.6971) -> (-7.7261, -14.0121) centre (0, 0) ccw
  arc A89 (-0.1738, -13.7489) -> (-0.5763, -14.1044) centre (-0.1788, -14.1489) ccw
  spline S89 degree 3 poles (-10.3836, -10.2786) (-10.5532, -10.5719) (-10.7651, -11.0274) (-10.9388, -11.678) knots 0 0 0 0 1 1 1 1
  arc A90 (0.5763, -14.1044) -> (0.1738, -13.7489) centre (0.1788, -14.1489) ccw
  spline S90 degree 3 poles (0.5763, -14.1044) (0.5816, -14.1594) (0.6033, -14.3245) (0.6905, -14.5943) knots 0 0 0 0 1 1 1 1
  spline S91 degree 3 poles (0.6905, -14.5943) (0.795, -14.9166) (0.9916, -15.3788) (1.3589, -15.9432) knots 0 0 0 0 1 1 1 1
  spline S92 degree 3 poles (-15.9979, -0.315) (-15.3982, -0.6213) (-14.9179, -0.7686) (-14.5865, -0.8388) knots 0 0 0 0 1 1 1 1
  arc A91 (-11.9266, -7.5514) -> (-11.82, -7.025) centre (-12.1639, -7.2293) ccw
  arc A92 (-14.743, -6.2191) -> (-14.4867, -6.7947) centre (0, 0) ccw
  spline S93 degree 3 poles (-7.7261, -14.0121) (-7.161, -13.6459) (-6.7933, -13.3036) (-6.5668, -13.0517) knots 0 0 0 0 1 1 1 1
  arc A93 (-13.6554, 1.61) -> (-13.6917, 1.2643) centre (0, 0) ccw
  spline S94 degree 3 poles (-15.5828, -3.6343) (-14.9325, -3.8092) (-14.4321, -3.8534) (-14.0933, -3.8532) knots 0 0 0 0 1 1 1 1
  arc A94 (-13.1297, -4.0834) -> (-13.0223, -4.4139) centre (0, 0) ccw
  spline S95 degree 3 poles (-13.236, -4.9067) (-13.2867, -4.9286) (-13.437, -5.0003) (-13.6666, -5.1666) knots 0 0 0 0 1 1 1 1
  spline S96 degree 3 poles (-12.9842, -6.6992) (-12.707, -6.6398) (-12.5532, -6.576) (-12.503, -6.5531) knots 0 0 0 0 1 1 1 1
  arc A95 (-13.236, -4.9067) -> (-13.0223, -4.4139) centre (-13.4011, -4.5423) ccw
  arc A96 (-10.3337, -9.0707) -> (-10.8673, -9.0094) centre (-10.6343, -9.3345) ccw
  spline S97 degree 3 poles (-6.5668, -13.0517) (-6.3774, -12.8407) (-6.2905, -12.6987) (-6.2633, -12.6506) knots 0 0 0 0 1 1 1 1
  arc A97 (-5.2103, -13.1195) -> (-5.4334, -12.6309) centre (-5.5915, -12.9984) ccw
  arc A98 (-5.2432, -15.1176) -> (-4.644, -15.3123) centre (0, 0) ccw
  spline S98 degree 3 poles (-11.3077, -9.2524) (-11.0489, -9.1366) (-10.9117, -9.0423) (-10.8673, -9.0094) knots 0 0 0 0 1 1 1 1
  spline S99 degree 3 poles (-5.3052, -13.6134) (-5.3409, -13.9503) (-5.3492, -14.4526) (-5.2432, -15.1176) knots 0 0 0 0 1 1 1 1
  arc A99 (-5.7509, -12.4896) -> (-6.2633, -12.6506) centre (-5.9182, -12.8529) ccw
  spline S100 degree 3 poles (-2.3687, -13.9161) (-2.375, -13.9709) (-2.3881, -14.1369) (-2.3589, -14.4189) knots 0 0 0 0 1 1 1 1
  arc A100 (-10.096, -9.866) -> (-10.1011, -9.329) centre (-10.395, -9.6003) ccw
  spline S101 degree 3 poles (-1.3589, -15.9432) (-0.9916, -15.3788) (-0.795, -14.9166) (-0.6905, -14.5943) knots 0 0 0 0 1 1 1 1
  spline S102 degree 3 poles (-2.3589, -14.4189) (-2.3237, -14.7559) (-2.2275, -15.2489) (-1.9855, -15.8773) knots 0 0 0 0 1 1 1 1
  arc A101 (-10.9388, -11.678) -> (-10.4706, -12.0996) centre (0, 0) ccw
  arc A102 (-5.7509, -12.4896) -> (-5.4334, -12.6309) centre (0, 0) ccw
  spline S103 degree 3 poles (-4.644, -15.3123) (-4.1674, -14.8366) (-3.8789, -14.4253) (-3.7097, -14.1318) knots 0 0 0 0 1 1 1 1
  arc A103 (-3.0285, -13.4123) -> (-3.4962, -13.6764) centre (-3.1166, -13.8025) ccw
  arc A104 (-13.6917, -1.2643) -> (-13.6554, -1.61) centre (0, 0) ccw
  arc A105 (-11.9938, -6.7239) -> (-12.503, -6.5531) centre (-12.3427, -6.9196) ccw
  spline S104 degree 3 poles (-13.9669, -2.0475) (-14.0211, -2.0585) (-14.183, -2.0973) (-14.4421, -2.2122) knots 0 0 0 0 1 1 1 1
  spline S105 degree 3 poles (-10.096, -9.866) (-10.1333, -9.9067) (-10.2415, -10.0333) (-10.3836, -10.2786) knots 0 0 0 0 1 1 1 1
  spline S106 degree 3 poles (-14.4867, -6.7947) (-13.8143, -6.8306) (-13.3156, -6.7698) (-12.9842, -6.6992) knots 0 0 0 0 1 1 1 1
  spline S107 degree 3 poles (-9.1369, -11.4012) (-8.9078, -11.2342) (-8.7932, -11.1134) (-8.7567, -11.072) knots 0 0 0 0 1 1 1 1
  arc A106 (-15.7138, -3.018) -> (-15.5828, -3.6343) centre (0, 0) ccw
  arc A107 (-11.9938, -6.7239) -> (-11.82, -7.025) centre (0, 0) ccw
  arc A108 (-10.3337, -9.0707) -> (-10.1011, -9.329) centre (0, 0) ccw
  spline S108 degree 3 poles (-12.2938, -7.8951) (-12.5206, -8.1467) (-12.8226, -8.5482) (-13.1278, -9.1485) knots 0 0 0 0 1 1 1 1
  arc A109 (-7.8241, -11.7495) -> (-7.9408, -11.2252) centre (-8.1718, -11.5518) ccw
  arc A110 (-8.222, -11.0209) -> (-8.7567, -11.072) centre (-8.4612, -11.3416) ccw
  spline S109 degree 3 poles (-14.4421, -2.2122) (-14.7517, -2.3498) (-15.1909, -2.5937) (-15.7138, -3.018) knots 0 0 0 0 1 1 1 1
  spline S110 degree 3 poles (-13.6666, -5.1666) (-13.9408, -5.3655) (-14.3197, -5.6954) (-14.743, -6.2191) knots 0 0 0 0 1 1 1 1
  spline S111 degree 3 poles (-5.2103, -13.1195) (-5.2279, -13.1718) (-5.2752, -13.3315) (-5.3052, -13.6134) knots 0 0 0 0 1 1 1 1
  spline S112 degree 3 poles (-3.7097, -14.1318) (-3.5684, -13.8861) (-3.5128, -13.7291) (-3.4962, -13.6764) knots 0 0 0 0 1 1 1 1
  spline S113 degree 3 poles (-0.6905, -14.5943) (-0.6033, -14.3245) (-0.5816, -14.1594) (-0.5763, -14.1044) knots 0 0 0 0 1 1 1 1
  spline S114 degree 3 poles (1.9855, -15.8773) (2.2275, -15.2489) (2.3237, -14.7559) (2.3589, -14.4189) knots 0 0 0 0 1 1 1 1
  arc A111 (1.3589, -15.9432) -> (1.9855, -15.8773) centre (0, 0) ccw
  arc A112 (-0.1738, -13.7489) -> (0.1738, -13.7489) centre (0, 0) ccw
  arc A113 (6.2633, -12.6506) -> (5.7509, -12.4896) centre (5.9182, -12.8529) ccw
  spline S115 degree 3 poles (5.3052, -13.6134) (5.2752, -13.3315) (5.2279, -13.1718) (5.2103, -13.1195) knots 0 0 0 0 1 1 1 1
  arc A114 (5.4334, -12.6309) -> (5.2103, -13.1195) centre (5.5915, -12.9984) ccw
  arc A115 (5.4334, -12.6309) -> (5.7509, -12.4896) centre (0, 0) ccw
  arc A116 (7.7261, -14.0121) -> (8.2718, -13.6971) centre (0, 0) ccw
  spline S116 degree 3 poles (6.2633, -12.6506) (6.2905, -12.6987) (6.3774, -12.8407) (6.5668, -13.0517) knots 0 0 0 0 1 1 1 1
  spline S117 degree 3 poles (6.5668, -13.0517) (6.7933, -13.3036) (7.161, -13.6459) (7.7261, -14.0121) knots 0 0 0 0 1 1 1 1
  arc A117 (7.9408, -11.2252) -> (8.222, -11.0209) centre (0, 0) ccw
  spline S118 degree 3 poles (8.2718, -13.6971) (8.2372, -13.0246) (8.1246, -12.535) (8.0197, -12.2129) knots 0 0 0 0 1 1 1 1
  arc A118 (7.9408, -11.2252) -> (7.8241, -11.7495) centre (8.1718, -11.5518) ccw
  arc A119 (8.7567, -11.072) -> (8.222, -11.0209) centre (8.4612, -11.3416) ccw
  spline S119 degree 3 poles (5.2432, -15.1176) (5.3492, -14.4526) (5.3409, -13.9503) (5.3052, -13.6134) knots 0 0 0 0 1 1 1 1
extrude "Extrude1" add sketch "sketch 24713" along normal blind 7.5 in component "Spur Gear (30 teeth)"
sketch "Sketch1" plane through (0, 0, 0) normal (0, 1, 0) x (1, 0, 0) in component "Spur Gear (30 teeth)"
  circle A0 centre (0, 0) radius 15 construction
component "Spur Gear (30 teeth)" placed x (1, 0, 0) y (0, 1, 0) z (0, 0, 1) at (0, 0, 0)
